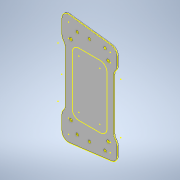
# Autodesk Inventor part: ChargerHolder
Saved by Autodesk Inventor 2021 (Build 250183000, 183)
## iProperties
Created: 2021-02-10
Part Number: ChargerHolder
Material: Generic
Document SubType Name: Modeling
Designer: Viktor
Density: 1 g/cm^3
Appearance: Default
Author: Viktor
Autodesk Inventor part; units mm, degrees
ref_plane "YZ Plane" through (0, 0, 0) normal (1, 0, 0) x (0, 1, 0)
ref_plane "XZ Plane" through (0, 0, 0) normal (0, 1, 0) x (-1, 0, 0)
ref_plane "XY Plane" through (0, 0, 0) normal (0, 0, 1) x (1, 0, 0)
sketch "Sketch1" plane through (0, 0, 0) normal (0, 0, 1) x (1, 0, 0)
  line L0 (0, 162.5) -> (0, -162.5)
  line L1 (0, -162.5) -> (160, -142.5)
  line L2 (160, -142.5) -> (160, 142.5)
  line L3 (160, 142.5) -> (0, 162.5)
  point P0 (0, 0)
  dimension "d0" = 285
  dimension "d1" = 325
  dimension "d2" = 162.5
  dimension "d3" = 142.5
  dimension "d4" = 160
  constraints: 8 end point, 1 midpoint, 1 vertical
  measures "d0" distance of L1.end L2.end
  measures "d1" distance of L0.start L0.end
  measures "d2" distance of L0.end point (0, 0)
  measures "d3" vertical distance of point (0, 0) L2.end
  measures "d4" distance between parallel lines of L2 L0
extrude "Extrusion1" add sketch "Sketch1" along normal blind 3
fillet "Fillet1" radius 20 4 edges at (160, 142.5, 1.5) (0, 162.5, 1.5) (0, -162.5, 1.5) (160, -142.5, 1.5)
sketch "Sketch2" plane through (0, 0, 3) normal (0, 0, 1) x (1, 0, 0)
  line L0 (-46, 0) -> (206, 0) projected
  line L1 (130, -90) -> (30, -90)
  line L2 (30, -90) -> (30, 90)
  line L3 (30, 90) -> (130, 90)
  line L4 (130, 90) -> (130, -90)
  line L5 (130, -90) -> (30, 90) construction
  line L6 (30, -90) -> (130, 90) construction
  line L7 (0, 139.8444) -> (0, -139.8444) projected
  line L8 (10, -90) -> (0, -90)
  line L9 (0, -90) -> (0, 90)
  line L10 (0, 90) -> (10, 90)
  line L11 (10, 90) -> (10, -90)
  line L12 (10, -90) -> (0, 90) construction
  line L13 (0, -90) -> (10, 90) construction
  line L14 (160, -124.8444) -> (160, 124.8444) projected
  line L15 (150, -90) -> (160, -90)
  line L16 (160, -90) -> (160, 90)
  line L17 (160, 90) -> (150, 90)
  line L18 (150, 90) -> (150, -90)
  line L19 (150, -90) -> (160, 90) construction
  line L20 (160, -90) -> (150, 90) construction
  point P0 (0, 0)
  point P1 (80, 0)
  point P2 (5, 0)
  point P3 (155, 0)
  point P4 (0, -90)
  dimension "d8" = 100
  dimension "d9" = 30
  dimension "d10" = 180
  dimension "d17" = 10
  dimension "d18" = 10
  constraints: 36 end point, 7 midpoint, 6 parallel, 6 point on line, 3 horizontal, 3 perpendicular
  measures "d8" distance between parallel lines of L4 L2
  measures "d9" distance between parallel lines of L7 L2
  measures "d10" distance between parallel lines of L3 L1
  measures "d17" distance between parallel lines of L7 L11
  measures "d18" distance between parallel lines of L16 L18
extrude "Extrusion2" cut sketch "Sketch2" against normal through all
fillet "Fillet2" radius 20 4 edges at (30, -90, 1.5) (130, -90, 1.5) (130, 90, 1.5) (30, 90, 1.5)
fillet "Fillet3" radius 20 8 edges at (10, -90, 1.5) (0, -90, 1.5) (10, 90, 1.5) (0, 90, 1.5) (150, 90, 1.5) (160, 90, 1.5) (150, -90, 1.5) (160, -90, 1.5)
sketch "Sketch4" plane through (0, 0, 3) normal (0, 0, 1) x (1, 0, 0)
  circle A0 centre (27, -100.5) radius 3.25
  line L0 (80.5, -98.3586) -> (80.5, 89.1662) construction
  line L1 (-46, 0) -> (206, 0) construction
  circle A1 centre (134, -100.5) radius 3.25
  circle A2 centre (27, 100.5) radius 3.25
  circle A3 centre (134, 100.5) radius 3.25
  point P0 (0, 0)
  point P1 (80.5, 98.3586)
  dimension "d20" = 6.5
  dimension "d21" = 100.5
  dimension "d22" = 107
  constraints: 4 centre point, 4 symmetric about line, 2 end point, 1 vertical, 3 other
  measures "d20" diameter of A0
  measures "d21" distance from line of L1 A0.centre
  measures "d22" distance of A1.centre A0.centre
extrude "Extrusion3" cut sketch "Sketch4" against normal blind 6
sketch "Sketch5" plane through (0, 0, 3) normal (0, 0, 1) x (1, 0, 0)
  circle A0 centre (125, -127.5) radius 2.75
  line L0 (160, -124.8444) -> (160, -99.137) projected
  line L1 (125, -127.5) -> (-64, -127.5) construction
  circle A1 centre (80, -127.5) radius 2.75
  circle A2 centre (45, -127.5) radius 2.75
  line L2 (-110.8, 0) -> (216.8, 0) projected
  circle A3 centre (125, 127.5) radius 2.75
  circle A4 centre (80, 127.5) radius 2.75
  circle A5 centre (45, 127.5) radius 2.75
  point P0 (0, 0)
  dimension "d25" = 5.5
  dimension "d26" = 35
  dimension "d27" = 80
  dimension "d28" = 115
  dimension "d29" = 5.5
  dimension "d30" = 5.5
  dimension "d31" = 127.5
  constraints: 6 centre point, 3 symmetric about line, 2 end point, 2 point on line, 1 horizontal, 3 other
  measures "d25" diameter of A0
  measures "d26" distance from line of L0 L1.start
  measures "d27" distance from line of L0 A1.centre
  measures "d28" distance from line of L0 A2.centre
  measures "d29" diameter of A2
  measures "d30" diameter of A1
  measures "d31" distance from line of point (0, 0) L1
extrude "Extrusion4" cut sketch "Sketch5" against normal through all
sketch "Sketch6" plane through (0, 0, 3) normal (0, 0, 1) x (1, 0, 0)
  circle A0 centre (125, -127.5) radius 2.75 projected
  circle A1 centre (125, 127.5) radius 2.75 projected
  circle A2 centre (80, -127.5) radius 2.75 projected
  circle A3 centre (45, 127.5) radius 2.75 projected
  circle A4 centre (80, 127.5) radius 2.75 projected
  circle A5 centre (45, -127.5) radius 2.75 projected
  circle A6 centre (27, 100.5) radius 3.25 projected
  circle A7 centre (134, -100.5) radius 3.25 projected
  circle A8 centre (134, 100.5) radius 3.25 projected
  circle A9 centre (27, -100.5) radius 3.25 projected
  arc A10 (160, -99.137) -> (155, -85.9082) centre (140, -99.137) ccw projected
  arc A11 (150, -72.6795) -> (155, -85.9082) centre (170, -72.6795) ccw projected
  line L0 (150, -72.6795) -> (150, 72.6795) projected
  arc A12 (155, 85.9082) -> (150, 72.6795) centre (170, 72.6795) ccw projected
  arc A13 (155, 85.9082) -> (160, 99.137) centre (140, 99.137) ccw projected
  line L1 (160, 99.137) -> (160, 124.8444) projected
  arc A14 (160, 124.8444) -> (142.4807, 144.6899) centre (140, 124.8444) ccw projected
  line L2 (142.4807, 144.6899) -> (22.4807, 159.6899) projected
  arc A15 (22.4807, 159.6899) -> (0, 139.8444) centre (20, 139.8444) ccw projected
  line L3 (0, 139.8444) -> (0, 99.137) projected
  arc A16 (0, 99.137) -> (5, 85.9082) centre (20, 99.137) ccw projected
  arc A17 (10, 72.6795) -> (5, 85.9082) centre (-10, 72.6795) ccw projected
  line L4 (10, 72.6795) -> (10, -72.6795) projected
  arc A18 (5, -85.9082) -> (10, -72.6795) centre (-10, -72.6795) ccw projected
  arc A19 (5, -85.9082) -> (0, -99.137) centre (20, -99.137) ccw projected
  line L5 (0, -99.137) -> (0, -139.8444) projected
  arc A20 (0, -139.8444) -> (22.4807, -159.6899) centre (20, -139.8444) ccw projected
  line L6 (22.4807, -159.6899) -> (142.4807, -144.6899) projected
  arc A21 (142.4807, -144.6899) -> (160, -124.8444) centre (140, -124.8444) ccw projected
  line L7 (160, -124.8444) -> (160, -99.137) projected
  line L8 (50, 90) -> (110, 90) projected
  arc A22 (130, 70) -> (110, 90) centre (110, 70) ccw projected
  line L9 (130, 70) -> (130, -70) projected
  arc A23 (110, -90) -> (130, -70) centre (110, -70) ccw projected
  line L10 (110, -90) -> (50, -90) projected
  arc A24 (30, -70) -> (50, -90) centre (50, -70) ccw projected
  line L11 (30, -70) -> (30, 70) projected
  arc A25 (50, 90) -> (30, 70) centre (50, 70) ccw projected
  point P0 (0, 0)
sketch "Sketch7" plane through (0, 0, 0) normal (0, 0, -1) x (-1, 0, 0)
  arc A0 (-130, -70) -> (-110, -90) centre (-110, -70) ccw projected
  line L0 (-130, -70) -> (-130, 70) projected
  arc A1 (-110, 90) -> (-130, 70) centre (-110, 70) ccw projected
  line L1 (-110, 90) -> (-50, 90) projected
  arc A2 (-30, 70) -> (-50, 90) centre (-50, 70) ccw projected
  line L2 (-30, 70) -> (-30, -70) projected
  arc A3 (-50, -90) -> (-30, -70) centre (-50, -70) ccw projected
  line L3 (-50, -90) -> (-110, -90) projected
  point P0 (0, 0)
extrude "Extrusion5" add sketch "Sketch7" against normal up to surface (3 mm away)
chamfer "Chamfer1" distance 1 angle 45 30 edges at (158.7083, 92.0659, 3) (158.7083, -92.0659, 3) (160, -111.9907, 3) (154.9936, -138.0804, 3) (82.4807, -152.1899, 3) (6.7639, -154.8379, 3) (0, -119.4907, 3) (1.2917, 92.0659, 3) (1.2917, -92.0659, 3) (8.7083, 79.7506, 3) (8.7083, -79.7506, 3) (10, 0, 3) (0, 119.4907, 3) (6.7639, 154.8379, 3) (82.4807, 152.1899, 3) (154.9936, 138.0804, 3) (160, 111.9907, 3) (151.2917, 79.7506, 3) (151.2917, -79.7506, 3) (150, 0, 3) (122.25, -127.5, 3) (77.25, -127.5, 3) (42.25, -127.5, 3) (23.75, -100.5, 3) (130.75, -100.5, 3) (130.75, 100.5, 3) (122.25, 127.5, 3) (77.25, 127.5, 3) (42.25, 127.5, 3) (23.75, 100.5, 3)
equation "\"d2\" = 0.5 * d1"
equation "\"d3\" = 0.5 * d0"
equation "\"d29\" = d25"
equation "\"d30\" = d25"
body "Solid1"
